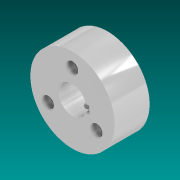
# Autodesk Inventor part: spiebaan mount 10 mm
Saved by Autodesk Inventor 2020.3 (Build 243373000, 373)
## iProperties
Created: 2020-05-22
Part Number: spiebaan mount 10 mm
Material: Aluminum 6061
Document SubType Name: Modeling
Designer: Svend
Density: 2.7 g/cm^3
Appearance: Aluminum - Polished
Author: Svend
Autodesk Inventor part; units mm, degrees
ref_plane "YZ Plane" through (0, 0, 0) normal (1, 0, 0) x (0, 1, 0)
ref_plane "XY Plane" through (0, 0, 0) normal (0, 0, 1) x (1, 0, 0)
sketch "Sketch1" plane through (0, 0, 0) normal (0, 0, 1) x (1, 0, 0)
  circle A0 centre (0, 0) radius 12
  circle A1 centre (0, 0) radius 4
  line L0 (3.873, 1) -> (4.8, 1)
  line L1 (4.8, 1) -> (4.8, -1)
  line L2 (4.8, -1) -> (3.873, -1)
  circle A2 centre (0, 8) radius 2
  circle A3 centre (-6.9282, -4) radius 2
  circle A4 centre (6.9282, -4) radius 2
  point P0 (4.8, 0)
  point P1 (-4, 0)
  dimension "d0" = 24
  dimension "d1" = 8
  dimension "d2" = 2
  dimension "d3" = 8.8
  dimension "d4" = 4
  dimension "d5" = 8
  dimension "d8" = 360
  constraints: 6 end point, 5 centre point, 3 point on circle, 2 coincident, 2 horizontal alignment, 2 perpendicular, 1 horizontal, 1 midpoint, 1 vertical alignment, 7 other
  measures "d0" diameter of A0
  measures "d1" diameter of A1
  measures "d2" distance between parallel lines of L2 L0
  measures "d3" distance of point (-4, 0) point (4.8, 0)
  measures "d4" diameter of A2
  measures "d5" distance of point (0, 0) A2.centre
extrude "Extrusion1" add sketch "Sketch1" along normal blind 10 contours A0 | A2 | A3 | A4
ref_plane "Work Plane3" through (0, 0, 0) normal (0, 1, 0) x (0, 0, 1)
ref_plane "Work Plane2" through (0, 0, 0) normal (0.866, -0.5, 0) x (0, 0, 1)
sketch "Sketch2" plane through (0, 0, 0) normal (0, 1, 0) x (0, 0, 1)
  line L0 (10, -12) -> (10, 12) projected
  line L1 (0, -12) -> (0, 12) projected
  line L2 (0, 12) -> (10, 12) projected
  line L3 (0, -12) -> (10, -12) projected
  point P0 (0, 0)
  point P1 (5, 0)
  point P2 (5, -12)
  point P3 (10, 0)
  constraints: 2 midpoint, 1 horizontal alignment, 1 vertical alignment
hole "Hole1" at (0, 0, 5) direction (0, -1, 0) diameter 2.459 end through all thread size "M3x0.5" class "6H" standard "ISO Metric profile"
sketch "Sketch3" plane through (0, 0, 0) normal (0.866, -0.5, 0) x (0, 0, 1)
  line L0 (0, -12) -> (0, 12) projected
  line L1 (0, -3.266) -> (0, -1.534) projected
  line L2 (0, -2.8025) -> (0, -3.266) projected
  line L3 (0, -1.0705) -> (0, -2.8025) projected
  line L4 (0, -1.534) -> (0, -1.0705) projected
  line L5 (0, 12) -> (10, 12) projected
  line L6 (0, -12) -> (10, -12) projected
  point P0 (0, 0)
  point P1 (0, 2)
  point P2 (0, -2)
  point P3 (0, 8.9282)
  point P4 (0, 4.9282)
  point P5 (0, -4.9282)
  point P6 (0, -8.9282)
  point P7 (5, 0)
  point P8 (5, -12)
  point P9 (0, 0)
  constraints: 2 midpoint, 1 horizontal alignment, 1 vertical alignment
hole "Hole2" at (0, 0, 5) direction (-0.866, 0.5, 0) diameter 2.459 end through all thread size "M3x0.5" class "6H" standard "ISO Metric profile"
hole "Hole3" at (0, 8, 0) at (-6.9282, -4, 0) at (6.9282, -4, 0) direction (0, 0, 1) diameter 3.242 end through all thread size "M4x0.7" class "6H" standard "ISO Metric profile"
ref_plane "Work Plane1" through (0, 0, 0) normal (-0.5, -0.866, 0) x (0, 0, 1)
body "Solid1"
